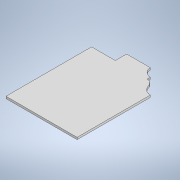
# Autodesk Inventor part: Base Drawing
Saved by Autodesk Inventor 2020 (Build 240168000, 168)
## iProperties
Created: 2020-04-06
Part Number: Base Drawing
Material: Generic
Document SubType Name: Modeling
Designer: Thomas J H Dodd
Density: 1 g/cm^3
Appearance: Default
Author: Thomas J H Dodd
Autodesk Inventor part; units mm, degrees
ref_plane "YZ Plane" through (0, 0, 0) normal (1, 0, 0) x (0, 1, 0)
ref_plane "XZ Plane" through (0, 0, 0) normal (0, 1, 0) x (-1, 0, 0)
ref_plane "XY Plane" through (0, 0, 0) normal (0, 0, 1) x (1, 0, 0)
sketch "Sketch1" plane through (0, 0, 0) normal (0, 1, 0) x (-1, 0, 0)
  line L0 (0, 0) -> (0, -415)
  line L1 (0, -415) -> (-115, -415)
  line L2 (-115, -415) -> (-115, -470)
  line L3 (-115, -470) -> (-230, -470)
  line L4 (-230, -470) -> (-345, -470) construction
  line L5 (0, 0) -> (-345, 0)
  line L6 (-345, 0) -> (-345, -355)
  line L7 (-270, -415) -> (-270, -430)
  arc A0 (-230, -470) -> (-270, -430) centre (-270.8018, -470.8018) ccw
  line L8 (-345, -355) -> (-345, -360) construction
  line L9 (-345, -360) -> (-325, -360) construction
  line L10 (-345, -360) -> (-345, -365) construction
  line L11 (-345, -365) -> (-345, -370) construction
  line L12 (-345, -370) -> (-345, -375) construction
  line L13 (-345, -375) -> (-345, -380) construction
  line L14 (-345, -365) -> (-317, -365) construction
  line L15 (-345, -370) -> (-312, -370) construction
  line L16 (-345, -375) -> (-309, -375) construction
  line L17 (-345, -380) -> (-306, -380) construction
  line L18 (-345, -380) -> (-345, -385) construction
  line L19 (-345, -385) -> (-345, -390) construction
  line L20 (-345, -390) -> (-345, -395) construction
  line L21 (-345, -395) -> (-345, -400) construction
  line L22 (-345, -400) -> (-345, -405) construction
  line L23 (-345, -405) -> (-345, -410) construction
  line L24 (-345, -385) -> (-303, -385) construction
  line L25 (-345, -390) -> (-301, -390) construction
  line L26 (-345, -395) -> (-299, -395) construction
  line L27 (-345, -400) -> (-296, -400) construction
  line L28 (-345, -405) -> (-292, -405) construction
  line L29 (-345, -410) -> (-286, -410) construction
  arc A1 (-292, -405) -> (-270, -415) centre (-268.9, -383.38) ccw
  arc A2 (-299, -395) -> (-292, -405) centre (-258.5, -374.1) ccw
  arc A3 (-299, -395) -> (-317, -365) centre (-378, -422) ccw
  arc A4 (-317, -365) -> (-345, -355) centre (-346.4167, -403.1667) ccw
  dimension "d0" = 415
  dimension "d1" = 115
  dimension "d2" = 55
  dimension "d3" = 115
  dimension "d4" = 115
  dimension "d5" = 345
  dimension "d6" = 355
  dimension "d7" = 15
  dimension "d8" = 155
  dimension "d9" = 40
  dimension "d17" = 5
  dimension "d18" = 20
  dimension "d19" = 5
  dimension "d20" = 5
  dimension "d21" = 5
  dimension "d22" = 5
  dimension "d23" = 28
  dimension "d24" = 33
  dimension "d25" = 36
  dimension "d26" = 39
  dimension "d27" = 5
  dimension "d28" = 5
  dimension "d29" = 5
  dimension "d30" = 5
  dimension "d31" = 5
  dimension "d32" = 5
  dimension "d34" = 42
  dimension "d35" = 44
  dimension "d36" = 46
  dimension "d37" = 49
  dimension "d38" = 53
  dimension "d39" = 59
  dimension "d43" = 62.5
  constraints: 60 end point, 14 point on circle, 12 horizontal, 5 centre point, 5 perpendicular, 2 vertical
  measures "d0" distance of L0.start L0.end
  measures "d1" distance of L0.end L1.end
  measures "d2" distance of L1.end L2.end
  measures "d3" distance of L2.end L3.end
  measures "d4" distance of L3.end L4.end
  measures "d5" distance of L0.start L5.end
  measures "d6" distance of L5.end L6.end
  measures "d7" distance of L7.start L7.end
  measures "d8" distance between parallel lines of L7 L2
  measures "d9" distance from line of L3 L7.end
  measures "d17" distance of L6.end L8.end
  measures "d18" distance of L8.end L9.end
  measures "d19" distance of L8.end L10.end
  measures "d20" distance of L10.end L11.end
  measures "d21" distance of L11.end L12.end
  measures "d22" distance of L12.end L13.end
  measures "d23" distance of L10.end L14.end
  measures "d24" distance of L11.end L15.end
  measures "d25" distance of L12.end L16.end
  measures "d26" distance of L13.end L17.end
  measures "d27" distance of L13.end L18.end
  measures "d28" distance of L18.end L19.end
  measures "d29" distance of L19.end L20.end
  measures "d30" distance of L20.end L21.end
  measures "d31" distance of L21.end L22.end
  measures "d32" distance of L22.end L23.end
  measures "d34" distance of L18.end L24.end
  measures "d35" distance of L19.end L25.end
  measures "d36" distance of L20.end L26.end
  measures "d37" distance of L21.end L27.end
  measures "d38" distance of L22.end L28.end
  measures "d39" distance of L23.end L29.end
extrude "Extrusion1" add sketch "Sketch1" along normal blind 10
body "Solid1"
